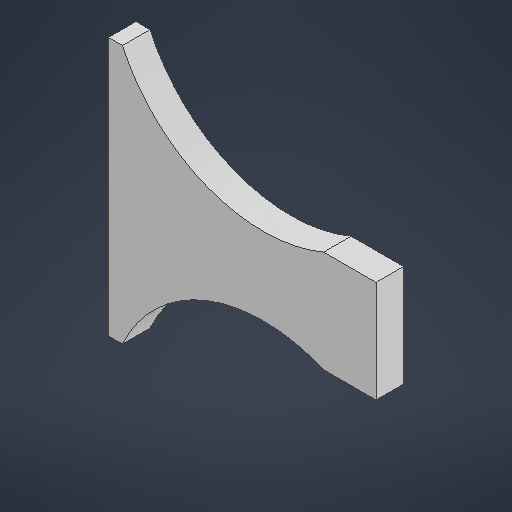
# Autodesk Inventor part: распорка
Saved by Autodesk Inventor 2025 (Build 290162000, 162)
## iProperties
Created: 2025-03-06
Part Number: распорка
Material: Типовые
Document SubType Name: Modeling
Designer: Phantom
Density: 1 g/cm^3
Appearance: По умолчанию
Author: Phantom
Autodesk Inventor part; units mm, degrees
ref_plane "YZ Plane" through (0, 0, 0) normal (1, 0, 0) x (0, 1, 0)
ref_plane "XZ Plane" through (0, 0, 0) normal (0, 1, 0) x (-1, 0, 0)
ref_plane "XY Plane" through (0, 0, 0) normal (0, 0, 1) x (1, 0, 0)
sketch "Эскиз1" plane through (0, 0, 0) normal (0, 0, 1) x (1, 0, 0)
  circle A0 centre (0, 0) radius 18
  line L0 (0, 0) -> (0, -45)
  circle A1 centre (0, -45) radius 18
  line L1 (13.0909, -12.3543) -> (13.0909, -32.6457)
  line L2 (-18, 0) -> (-18, -45)
  line L3 (10.0084, -14.961) -> (14.305, -14.961)
  line L4 (10.0084, -30.039) -> (17.305, -30.039)
  line L5 (-16.372, -7.4805) -> (-18, -7.4805)
  line L6 (-16.372, -37.5195) -> (-18, -37.5195)
  line L7 (7, -16.5831) -> (15.3551, -16.5831)
  line L8 (7, -28.4169) -> (18, -28.4169)
  point P0 (13.0909, -30.039)
  point P1 (13.0909, -14.961)
  point P2 (13.0909, -28.4169)
  point P3 (13.0909, -16.5831)
  dimension "d0" = 36
  dimension "d1" = 45
  dimension "d2" = 36
  constraints: 18 end point, 10 point on circle, 3 horizontal, 3 perpendicular, 3 point on line, 2 centre point, 2 coincident, 2 vertical, 1 tangent
  measures "d0" diameter of A0
  measures "d1" distance of L0.start L0.end
  measures "d2" diameter of A1
extrude "Выдавливание1" add sketch "Эскиз1" along normal blind 3.2 contours A0 L0 A1 L6 L2 L5 | A0 L7 L1 L8 A1 L0
